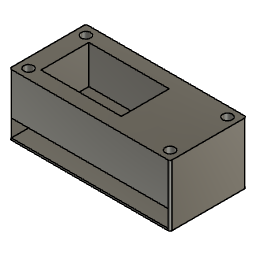
case v14 (Autodesk Fusion 360 design; units mm, degrees)
Autodesk Fusion 360 part; units mm, degrees
sketch "スケッチ1" plane through (0, 0, 0) normal (0, 0, 1) x (1, 0, 0)
  line L0 (0, 0) -> (84, 0)
  line L1 (84, 0) -> (84, 40)
  line L2 (84, 40) -> (0, 40)
  line L3 (0, 40) -> (0, 0)
  dimension "d1" = 40
  dimension "d2" = 84
  constraint horizontal L0
  constraint vertical L1
  constraint horizontal L2
  constraint vertical L3
  constraint coincident L0.start L3.end
  measures "d1" distance of L0.end L1.end
  measures "d2" distance of L0.start L0.end
extrude "押し出し1" add sketch "スケッチ1" along normal blind 32
sketch "スケッチ2" plane through (0, 0, 32) normal (0, 0, 1) x (-1, 0, 0)
  line L0 (0, -40) -> (0, 0)
  line L1 (0, 0) -> (-84, 0)
  line L2 (-84, 0) -> (-84, -40)
  line L3 (-84, -40) -> (0, -40)
  line L4 (-9, -32.5) -> (-51, -32.5)
  line L5 (-51, -32.5) -> (-51, -7.5)
  line L6 (-51, -7.5) -> (-9, -7.5)
  line L7 (-9, -7.5) -> (-9, -32.5)
  dimension "d5" = 42
  dimension "d6" = 25
  dimension "d27" = 9
  dimension "d72" = 7.5
  constraint horizontal L4
  constraint vertical L5
  constraint horizontal L6
  constraint vertical L7
  measures "d5" distance of L4.start L4.end
  measures "d6" distance of L4.end L5.end
  measures "d27" distance of L0 L7
  measures "d72" distance of L3 L4
extrude "押し出し2" cut sketch "スケッチ2" against normal blind 20 contours L4 L5 L6 L7
fillet "フィレット1" radius 1 4 edges at (84, 0, 16) (84, 40, 16) (0, 0, 16) (0, 40, 16)
sketch "スケッチ5" plane through (0, 0, 32) normal (0, 0, 1) x (-1, 0, 0)
  arc A0 (-1, -40) -> (0, -39) centre (-1, -39) ccw
  line L0 (0, -39) -> (0, -1)
  arc A1 (0, -1) -> (-1, 0) centre (-1, -1) ccw
  line L1 (-1, 0) -> (-83, 0)
  arc A2 (-83, 0) -> (-84, -1) centre (-83, -1) ccw
  line L2 (-84, -1) -> (-84, -39)
  arc A3 (-84, -39) -> (-83, -40) centre (-83, -39) ccw
  line L3 (-83, -40) -> (-1, -40)
  line L4 (-51, -32.5) -> (-51, -7.5)
  line L5 (-51, -7.5) -> (-9, -7.5)
  line L6 (-9, -7.5) -> (-9, -32.5)
  line L7 (-9, -32.5) -> (-51, -32.5)
  circle A4 centre (-5, -5) radius 2.5
  circle A5 centre (-5, -35) radius 2.5
  circle A6 centre (-79, -5) radius 2.5
  circle A7 centre (-79, -35) radius 2.5
  dimension "d28" = 5
  dimension "d29" = 5
  dimension "d30" = 5
  dimension "d31" = 5
  dimension "d32" = 5
  dimension "d33" = 5
  dimension "d34" = 5
  dimension "d35" = 5
  dimension "d36" = 5
  dimension "d37" = 5
  dimension "d38" = 5
  dimension "d39" = 5
  measures "d28" diameter of A4
  measures "d29" distance of L1 A4.centre
  measures "d30" distance of L0 A4.centre
  measures "d31" diameter of A5
  measures "d32" distance of L3 A5.centre
  measures "d33" distance of L0 A5.centre
  measures "d34" diameter of A6
  measures "d35" distance of L2 A6.centre
  measures "d36" distance of L1 A6.centre
  measures "d37" diameter of A7
  measures "d38" distance of L3 A7.centre
  measures "d39" distance of L2 A7.centre
extrude "押し出し4" cut sketch "スケッチ5" against normal blind 8 contours A4 | A5 | A6 | A7
sketch "スケッチ18" plane through (0, 0, 0) normal (0, -1, 0) x (1, 0, 0)
  line L0 (1, 32) -> (1, 0)
  line L1 (1, 0) -> (83, 0)
  line L2 (83, 0) -> (83, 32)
  line L3 (83, 32) -> (1, 32)
  line L4 (1, 1) -> (83, 1)
  line L5 (83, 1) -> (83, 10)
  line L6 (83, 10) -> (1, 10)
  line L7 (1, 10) -> (1, 1)
  dimension "d75" = 9
  constraint horizontal L4
  constraint vertical L5
  constraint horizontal L6
  constraint vertical L7
  constraint coincident L2 L5.end
  constraint coincident L0 L4.start
  measures "d75" distance of L4.start L6.end
extrude "押し出し16" cut sketch "スケッチ18" against normal blind 40 contours L0 L2 L4 L5 L6 L7
